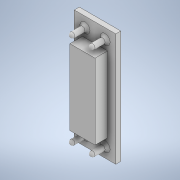
# Autodesk Inventor part: Long PDMS Chamber-Mold
Saved by Autodesk Inventor 2022 (Build 260153000, 153)
## iProperties
Created: 2021-04-09
Part Number: Long PDMS Chamber-Mold
Material: Generic
Document SubType Name: Modeling
Designer: Jeremy Hirota
Density: 1 g/cm^3
Appearance: Default
Author: Jeremy Hirota
Autodesk Inventor part; units mm, degrees
ref_plane "YZ Plane" through (0, 0, 0) normal (1, 0, 0) x (0, 1, 0)
ref_plane "XZ Plane" through (0, 0, 0) normal (0, 1, 0) x (-1, 0, 0)
ref_plane "XY Plane" through (0, 0, 0) normal (0, 0, 1) x (1, 0, 0)
sketch "Sketch1" plane through (0, 0, 0) normal (0, 0, 1) x (1, 0, 0)
  line L0 (-13.5, 42) -> (13.5, 42) construction
  line L1 (13.5, 42) -> (13.5, -42) construction
  line L2 (13.5, -42) -> (-13.5, -42) construction
  line L3 (-13.5, -42) -> (-13.5, 42) construction
  line L4 (-10, 30) -> (10, 30)
  line L5 (10, 30) -> (10, -30)
  line L6 (10, -30) -> (-10, -30)
  line L7 (-10, -30) -> (-10, 30)
  circle A0 centre (-8, 37) radius 2.025
  circle A1 centre (8, 37) radius 2.025
  circle A2 centre (8, -37) radius 2.025
  circle A3 centre (-8, -37) radius 2.025
  line L8 (-16.5, 45) -> (16.5, 45)
  line L9 (16.5, 45) -> (16.5, -45)
  line L10 (16.5, -45) -> (-16.5, -45)
  line L11 (-16.5, -45) -> (-16.5, 45)
  line L12 (-23.1, 0) -> (23.1, 0) projected
  point P0 (0, 0)
  dimension "d0" = 27
  dimension "d8" = 4.05
  dimension "d9" = 5
  dimension "d10" = 5.5
  dimension "d11" = 4.05
  dimension "d12" = 5.5
  dimension "d13" = 4.05
  dimension "d14" = 5
  dimension "d15" = 4.05
  dimension "d17" = 33
  dimension "d19" = 16.5
  dimension "d29" = 5.5
  dimension "d31" = 5
  dimension "d66" = 15
  dimension "d68" = 8
  dimension "d69" = 8
  dimension "d71" = 60
  dimension "d72" = 15
  dimension "d73" = 8
  dimension "d76" = 30
  dimension "d77" = 20
  dimension "d79" = 8
  constraints: 24 end point, 6 parallel, 4 centre point, 3 horizontal, 3 perpendicular
  measures "d0" distance of L1.end L2.end
  measures "d8" diameter of A0
  measures "d9" distance from line of L0 A0.centre
  measures "d10" distance from line of L3 A0.centre
  measures "d11" diameter of A1
  measures "d12" distance from line of L1 A1.centre
  measures "d13" diameter of A2
  measures "d14" distance from line of L2 A2.centre
  measures "d15" diameter of A3
  measures "d17" distance of L9.end L10.end
  measures "d19" distance from line of point (0, 0) L11
  measures "d29" distance from line of L3 A3.centre
  measures "d31" distance from line of L0 A1.centre
  measures "d66" distance between parallel lines of L10 L6
  measures "d68" distance from line of L10 A3.centre
  measures "d69" distance from line of L10 A2.centre
  measures "d71" distance of L4.end L5.end
  measures "d72" distance between parallel lines of L8 L4
  measures "d73" distance from line of L8 A0.centre
  measures "d76" distance between parallel lines of L12 L4
  measures "d77" distance of L5.end L6.end
  measures "d79" distance from line of L8 A1.centre
extrude "Extrusion1" add sketch "Sketch1" along normal blind 12 contours A0 | A1 | A2 | A3
extrude "Extrusion2" add sketch "Sketch1" against normal blind 4 contours L7 L12 L11 L8 L9 L5 L4 | L4 L5 L12 L7 | L12 L5 L6 L7 | L7 L6 L5 L12 L9 L10 L11 | A0 | A1 | A2 | A3
extrude "Extrusion3" [suppressed]
sketch "Sketch2" plane through (0, 0, 12) normal (0, 0, 1) x (1, 0, 0)
  line L0 (-10, -30) -> (10, -30) projected
  line L1 (10, -30) -> (10, 30) projected
  line L2 (10, 30) -> (-10, 30) projected
  line L3 (-10, 30) -> (-10, -30) projected
  circle A0 centre (-8, 37) radius 2.025 projected
  circle A1 centre (8, 37) radius 2.025 projected
  circle A2 centre (8, -37) radius 2.025 projected
  circle A3 centre (-8, -37) radius 2.025 projected
  point P0 (0, 0)
extrude "Extrusion4" [suppressed]
sketch "Sketch3" plane through (0, 0, -4) normal (0, 0, -1) x (-1, 0, 0)
  line L0 (31.5, 60) -> (-31.5, 60)
  line L1 (-31.5, 60) -> (-31.5, -60)
  line L2 (-31.5, -60) -> (31.5, -60)
  line L3 (31.5, -60) -> (31.5, 60)
  line L4 (16.5, -45) -> (16.5, 45) projected
  line L5 (-16.5, 45) -> (-16.5, -45) projected
  line L6 (-16.5, -45) -> (16.5, -45) projected
  line L7 (16.5, 45) -> (-16.5, 45) projected
  point P0 (0, 0)
  dimension "d32" = 15
  dimension "d33" = 15
  dimension "d34" = 15
  dimension "d35" = 15
  constraints: 8 end point, 2 parallel, 1 horizontal, 1 perpendicular
  measures "d32" distance between parallel lines of L4 L3
  measures "d33" distance between parallel lines of L5 L1
  measures "d34" distance between parallel lines of L6 L2
  measures "d35" distance between parallel lines of L7 L0
extrude "Extrusion5" [suppressed]
sketch "Sketch4" plane through (-31.5, -38, 0) normal (0, 0, 1) x (1, 0, 0)
  line L0 (0, 0) -> (0, 76) projected
  line L1 (0, 76) -> (63, 76) projected
  line L2 (0, 0) -> (63, 0)
  line L3 (63, 0) -> (63, 76)
  line L4 (63, 76) -> (0, 76)
  line L5 (0, 76) -> (0, 0)
  line L6 (60.5, 73.5) -> (2.5, 73.5)
  line L7 (2.5, 73.5) -> (2.5, 2.5)
  line L8 (2.5, 2.5) -> (60.5, 2.5)
  line L9 (60.5, 2.5) -> (60.5, 73.5)
  point P0 (31.5, 38)
  dimension "d38" = 2.5
  dimension "d39" = 2.5
  dimension "d40" = 2.5
  dimension "d41" = 2.5
  constraints: 16 end point, 4 parallel, 2 horizontal, 2 perpendicular
  measures "d38" distance between parallel lines of L1 L6
  measures "d39" distance between parallel lines of L3 L9
  measures "d40" distance between parallel lines of L2 L8
  measures "d41" distance between parallel lines of L0 L7
extrude "Extrusion6" [suppressed]
sketch "Sketch6" plane through (0, 0, -4) normal (0, 0, -1) x (-1, 0, 0)
  line L0 (-10, 30) -> (-10, -30) projected
  line L1 (10, -30) -> (-10, -30) projected
  line L2 (-10, 30) -> (10, 30)
  line L3 (10, 30) -> (10, -30)
  line L4 (10, -30) -> (-10, -30)
  line L5 (-10, -30) -> (-10, 30)
  point P0 (0, 0)
  constraints: 8 end point, 2 parallel, 1 horizontal, 1 perpendicular
extrude "Extrusion7" add sketch "Sketch6" against normal blind 14
sketch "Sketch7" plane through (0, 0, -4) normal (0, 0, -1) x (-1, 0, 0)
  circle A0 centre (8, -37) radius 2.025 projected
  circle A1 centre (8, -37) radius 2.1
  circle A2 centre (-8, -37) radius 2.025 projected
  circle A3 centre (-8, -37) radius 2.1
  circle A4 centre (-8, 37) radius 2.025 projected
  circle A5 centre (-8, 37) radius 2.1
  circle A6 centre (8, 37) radius 2.025 projected
  circle A7 centre (8, 37) radius 2.1
  point P0 (0, 0)
  dimension "d58" = 4.2
  dimension "d59" = 4.2
  dimension "d60" = 4.2
  dimension "d61" = 4.2
  constraints: 4 centre point, 4 coincident
  measures "d58" diameter of A1
  measures "d59" diameter of A3
  measures "d60" diameter of A5
  measures "d61" diameter of A7
extrude "Extrusion8" [suppressed]
fillet "Fillet1" [suppressed]
fillet "Fillet2" [suppressed]
fillet "Fillet3" radius 2 8 edges at (-10.025, -37, 12) (5.975, -37, 12) (5.975, 37, 12) (-10.025, 37, 12) (5.975, -37, 0) (-10.025, -37, 0) (5.975, 37, 0) (-10.025, 37, 0)
sketch "Sketch8" plane through (0, 0, 0) normal (0, 0, 1) x (1, 0, 0)
  point P0 (0, 0)
body "Solid1"
